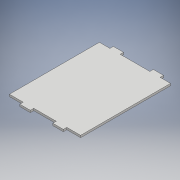
# Autodesk Inventor part: sideWall_r
Saved by Autodesk Inventor 2017 (Build 210142000, 142)
## iProperties
Created: 2017-06-02
Part Number: sideWall_r
Material: Generic
Document SubType Name: Modeling
Designer: Paolo
Density: 1 g/cm^3
Appearance: Default
Author: Paolo
Autodesk Inventor part; units mm, degrees
ref_plane "YZ Plane" through (0, 0, 0) normal (1, 0, 0) x (0, 1, 0)
ref_plane "XZ Plane" through (0, 0, 0) normal (0, 1, 0) x (-1, 0, 0)
ref_plane "XY Plane" through (0, 0, 0) normal (0, 0, 1) x (1, 0, 0)
sketch "Sketch1" plane through (0, 0, 0) normal (0, 0, 1) x (1, 0, 0)
  line L0 (0, -0.5) -> (15.6, -0.5) projected
  line L1 (0, -0.5) -> (0, -15) projected
  line L2 (0, -15) -> (15.6, -15) projected
  line L3 (15.6, -0.5) -> (15.6, -15) projected
  line L4 (47.8, -0.5) -> (63.4, -0.5) projected
  line L5 (47.8, -0.5) -> (47.8, -15) projected
  line L6 (47.8, -15) -> (63.4, -15) projected
  line L7 (63.4, -0.5) -> (63.4, -15) projected
  line L8 (53, 136.2) -> (53, 132.2) projected
  line L9 (53, 132.2) -> (68.2, 132.2) projected
  line L10 (68.2, 136.2) -> (68.2, 132.2) projected
  line L11 (68.2, 136.2) -> (53, 136.2) projected
  line L12 (-4.8, 136.2) -> (-4.8, 132.2) projected
  line L13 (-4.8, 132.2) -> (10.4, 132.2) projected
  line L14 (10.4, 136.2) -> (10.4, 132.2) projected
  line L15 (-4.8, 136.2) -> (10.4, 136.2) projected
  line L16 (63.2, -0.7) -> (48, -0.7)
  line L17 (48, -0.7) -> (48, -14.8)
  line L18 (48, -14.8) -> (63.2, -14.8)
  line L19 (63.2, -14.8) -> (63.2, -0.7)
  line L20 (15.4, -14.8) -> (0.2, -14.8)
  line L21 (0.2, -14.8) -> (0.2, -0.7)
  line L22 (0.2, -0.7) -> (15.4, -0.7)
  line L23 (15.4, -0.7) -> (15.4, -14.8)
  line L24 (53.2, 136) -> (53.2, 132.4)
  line L25 (53.2, 132.4) -> (68, 132.4)
  line L26 (68, 132.4) -> (68, 136)
  line L27 (68, 136) -> (53.2, 136)
  line L28 (10.2, 132.4) -> (-4.6, 132.4)
  line L29 (-4.6, 132.4) -> (-4.6, 136)
  line L30 (-4.6, 136) -> (10.2, 136)
  line L31 (10.2, 136) -> (10.2, 132.4)
  line L32 (-19.8, 130.2) -> (-19.8, 136.2) projected
  line L33 (-19.8, 130.2) -> (83.2, 130.2) projected
  line L34 (83.2, 136.2) -> (83.2, 130.2) projected
  line L35 (-19.8, 136.2) -> (83.2, 136.2) projected
  line L36 (-19.8, -29) -> (-19.8, 0) projected
  line L37 (-19.8, -29) -> (83.2, -29) projected
  line L38 (83.2, 0) -> (83.2, -29) projected
  line L39 (83.2, 0) -> (-19.8, 0) projected
  line L40 (67.8, -18.7754) -> (66.8, -18.7754) projected
  line L41 (66.8, -18.7754) -> (66.8, -22.0248) projected
  line L42 (66.8, -22.0248) -> (67.8, -22.0248) projected
  line L43 (67.8, -22.0248) -> (67.8, -24.6628) projected
  line L44 (67.8, -24.6628) -> (52.5, -24.6628) projected
  line L45 (52.5, -24.6628) -> (52.5, -22.0248) projected
  line L46 (52.5, -22.0248) -> (53.5, -22.0248) projected
  line L47 (53.5, -22.0248) -> (53.5, -18.7754) projected
  line L48 (53.5, -18.7754) -> (52.5, -18.7754) projected
  line L49 (52.5, -18.7754) -> (52.5, -16.1374) projected
  line L50 (52.5, -16.1374) -> (67.8, -16.1374) projected
  line L51 (67.8, -16.1374) -> (67.8, -18.7754) projected
  line L52 (-19.8, 130.2) -> (83.2, 130.2)
  line L53 (83.2, 130.2) -> (83.2, 0)
  line L54 (83.2, 0) -> (-19.8, 0)
  line L55 (-19.8, 0) -> (-19.8, 130.2)
  line L56 (63.2, -0.7) -> (63.2, 0)
  line L57 (48, -0.7) -> (48, 0)
  line L58 (15.4, -0.7) -> (15.4, 0)
  line L59 (0.2, -0.7) -> (0.2, 0)
  line L60 (0.2, -5) -> (15.4, -5)
  line L61 (48, -5) -> (63.2, -5)
  line L62 (53.2, 132.4) -> (53.2, 130.2)
  line L63 (68, 132.4) -> (68, 130.2)
  line L64 (10.2, 132.4) -> (10.2, 130.2)
  line L65 (-4.6, 132.4) -> (-4.6, 130.2)
  line L66 (-4.6, 135.2) -> (10.2, 135.2)
  line L67 (53.2, 135.2) -> (68, 135.2)
  point P0 (0, 0)
  dimension "d0" = 0.2
  dimension "d1" = 0.2
  dimension "d2" = 0.2
  dimension "d3" = 0.2
  dimension "d4" = 5
  dimension "d5" = 5
  constraints: 64 end point, 16 point on line, 11 perpendicular, 4 parallel, 2 collinear, 1 horizontal, 12 other
  measures "d0" distance between parallel lines of L4 L16
  measures "d1" distance between parallel lines of L3 L23
  measures "d2" distance between parallel lines of L11 L27
  measures "d3" distance between parallel lines of L14 L31
  measures "d4" distance between parallel lines of L60 L39
  measures "d5" distance between parallel lines of L33 L66
extrude "Extrusion1" add sketch "Sketch1" along normal blind 3 contours L59 L39 L58 L0 | L0 L58 L22 L59 | L22 L23 L60 L21 | L39 L55 L33 L53 | L39 L56 L4 L57 | L4 L56 L16 L57 | L65 L13 L64 L33 | L16 L19 L61 L17 | L65 L28 L64 L13 | L62 L9 L63 L33 | L29 L66 L31 L28 | L62 L25 L63 L9 | L24 L67 L26 L25
body "Solid1"
